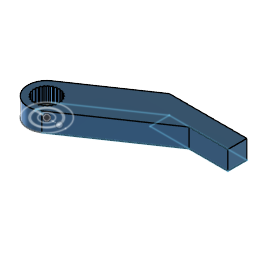
Box_Grils_Day (Autodesk Fusion 360 archive; units mm, degrees)
design "Bras  girls day v2"
Autodesk Fusion 360 part; units mm, degrees
sketch "Sketch1" plane through (0, 0, 0) normal (0, 0, 1) x (1, 0, 0)
  circle A0 centre (0, 0) radius 1.5
  circle A1 centre (0, 0) radius 2.75
  circle A2 centre (0, 0) radius 4.5
  circle A3 centre (0, 0) radius 3
  line L0 (0, 0) -> (-3, 0)
  line L1 (0, 0) -> (-2.9763, 0.376)
  line L2 (0, 0) -> (3, 0) construction
  line L3 (0, 0) -> (-2.906, 0.7452)
  line L4 (-2.9763, 0.376) -> (-2.6638, 0.6831)
  line L5 (-2.9763, 0.376) -> (-2.75, 0)
  line L6 (14.1674, 15.1142) -> (32.7197, 15.1142)
  line L7 (32.7197, 15.1142) -> (32.7197, 10.548)
  line L8 (32.7197, 10.548) -> (14.1674, 10.548)
  line L9 (14.1674, 10.548) -> (14.1674, 15.1142)
  line L10 (14.1674, 15.1142) -> (-2.5363, 3.7172)
  line L11 (2.5363, -3.7172) -> (23.4435, 10.548)
  dimension "d1" = 3
  dimension "d2" = 5.5
  dimension "d3" = 9
  dimension "d10" = 6
  dimension "d11" = 172.8
  dimension "d12" = 7.2
  constraint coincident A0.centre A1.centre
  constraint concentric A0 A2
  constraint coincident A3 L0.end
  constraint horizontal L0
  constraint horizontal L2
  constraint coincident A3 L3.end
  constraint coincident A1 L4.end
  constraint coincident L3 L4.end
  constraint coincident L0 L5.end
  constraint coincident A1 L5.end
  constraint horizontal L6
  constraint vertical L7
  constraint horizontal L8
  constraint vertical L9
  constraint coincident A2 L10.end
  constraint tangent A2 L10
  constraint coincident A2 L11.start
  constraint midpoint L8 L11.end
  constraint parallel L10 L11
  constraint tangent A2 L11
  measures "d1" diameter of A0
  measures "d2" diameter of A1
  measures "d3" diameter of A2
  measures "d10" diameter of A3
  measures "d11" angle of L1 L2
  measures "d12" angle of L0 L1
extrude "Extrude1" add sketch "Sketch1" along normal blind 1 contours A0 A1 L0 L3 | A0 A1 L1 L3 | A0 A1 L0 L1 makes body 1
extrude "Extrude2" add sketch "Sketch1" along normal blind 4.5 separate body contours A1 A3 L0 L3 | A3 L3 L4 | A1 L1 L4 | A1 L1 L5 | A3 L0 L5 | A2 makes body 2
extrude "Extrude3" add sketch "Sketch1" along normal blind 1 contours A0 A1 L0 L3 | A0 A1 L1 L3 | A0 A1 L0 L1 bodies 2
extrude "Extrude4" cut sketch "Sketch1" along normal blind 7 from surface at 1 contours A1 L1 L4 | A1 L1 L5 bodies 2
pattern_circular "C-Pattern1" count 25 over 360 about axis through (0, 0, 1.75) along (0, 0, 1) of "Extrude4"
extrude "Extrude5" add sketch "Sketch1" along normal blind 4.5 contours A2 L8 L9 L10 L11 | L6 L7 L8 L9 bodies 2
